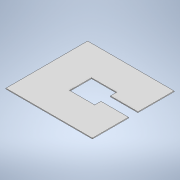
# Autodesk Inventor part: TopPaperCover
Saved by Autodesk Inventor 2022.3 (Build 263350000, 350)
## iProperties
Created: 2023-10-29
Part Number: TopPaperCover
Material: Generic
Document SubType Name: Modeling
Designer: Siggi
Density: 1 g/cm^3
Appearance: Default
Author: Siggi
Autodesk Inventor part; units mm, degrees
ref_plane "YZ Plane" through (0, 0, 0) normal (1, 0, 0) x (0, 1, 0)
ref_plane "XZ Plane" through (0, 0, 0) normal (0, 1, 0) x (-1, 0, 0)
ref_plane "XY Plane" through (0, 0, 0) normal (0, 0, 1) x (1, 0, 0)
sketch "Sketch1" plane through (0, 0, 0) normal (0, 1, 0) x (-1, 0, 0)
  line L0 (0, 0) -> (-110, 0)
  line L1 (-110, 104) -> (0, 104)
  line L2 (0, 104) -> (0, 0)
  line L3 (-110, 58) -> (-75, 58)
  line L4 (-75, 46) -> (-110, 46)
  line L5 (-110, 0) -> (-110, 46)
  line L6 (-110, 58) -> (-110, 104)
  line L7 (-75, 38) -> (-43, 38)
  line L8 (-43, 38) -> (-43, 66)
  line L9 (-43, 66) -> (-75, 66)
  line L10 (-75, 66) -> (-75, 58)
  line L11 (-75, 46) -> (-75, 38)
  dimension "d6" = 110
  dimension "d7" = 104
  dimension "d8" = 12
  dimension "d9" = 46
  dimension "d10" = 32
  dimension "d11" = 28
  dimension "d12" = 35
  constraints: 24 end point, 7 parallel, 3 horizontal, 3 perpendicular
  measures "d6" distance of L1.start L1.end
  measures "d7" distance of L1.end L0.start
  measures "d8" distance of L4.end L3.start
  measures "d9" distance of L3.start L1.start
  measures "d10" distance of L8.end L9.end
  measures "d11" distance of L7.end L8.end
  measures "d12" distance of L3.start L3.end
extrude "Extrusion1" add sketch "Sketch1" along normal blind 1
body "Solid1"
